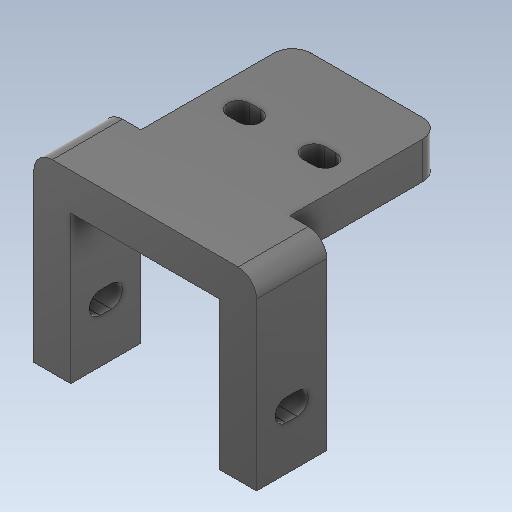
# Autodesk Inventor part: 0008-10-032 Suport cadru si axa Z
Saved by Autodesk Inventor 2020 (Build 240168000, 168)
## iProperties
Created: 2021-03-06
Part Number: 0008-10-032 Suport cadru si axa Z
Material: ABS Plastic
Document SubType Name: Modeling
Designer: Iulian Bors
Density: 1.06 g/cm^3
Appearance: Smooth - White
Mass: 43.4789 g
Surface Area: 130.984 cm^2
Volume: 41.0179 cm^3
Description: Suport cadru
Author: Iulian Bors
Subject: 032
Autodesk Inventor part; units mm, degrees
ref_plane "YZ Plane" through (0, 0, 0) normal (1, 0, 0) x (0, 1, 0)
ref_plane "XZ Plane" through (0, 0, 0) normal (0, 1, 0) x (-1, 0, 0)
ref_plane "XY Plane" through (0, 0, 0) normal (0, 0, 1) x (1, 0, 0)
sketch "Sketch1" plane through (0, 0, 0) normal (0, 0, 1) x (1, 0, 0)
  line L0 (-20.15, 20) -> (20.15, 20)
  line L1 (20.15, 20) -> (20.15, -20)
  line L2 (20.15, -20) -> (-20.15, -20)
  line L3 (-20.15, -20) -> (-20.15, 20)
  line L4 (30.15, 30) -> (-30.15, 30)
  line L5 (-30.15, 30) -> (-30.15, -30)
  line L6 (-30.15, -30) -> (30.15, -30)
  line L7 (30.15, -30) -> (30.15, 30)
  line L8 (-20.15, -20) -> (-30.15, -20)
  line L9 (20.15, -20) -> (30.15, -20)
  point P0 (0, 0)
  point P1 (0, 20)
  point P2 (-20.15, 0)
  dimension "d0" = 40.3
  dimension "d1" = 40
  dimension "d2" = 10
  constraints: 20 end point, 5 equal length, 3 perpendicular, 2 midpoint, 2 point on line, 1 horizontal, 1 horizontal alignment, 1 vertical alignment, 3 other
  measures "d0" distance of L0.start L0.end
  measures "d1" distance of L2.end L0.start
  measures "d2" distance between parallel lines of L0 L4
extrude "Extrusion1" add sketch "Sketch1" along normal blind 60 contours L3 L8 L5 L4 L7 L9 L1 L0
sketch "Sketch3" plane through (30.15, -20, 0) normal (1, 0, 0) x (0, 0, -1)
  line L0 (-41, 40) -> (0, 40)
  line L1 (0, 40) -> (0, 0)
  line L2 (0, 0) -> (-41, 0)
  line L3 (-41, 0) -> (-41, 40)
  line L4 (-60, 0) -> (-60, 50) projected
  line L5 (0, 0) -> (-60, 0) projected
  line L6 (0, 50) -> (-60, 50) projected
  line L7 (0, 0) -> (0, 50) projected
  point P0 (0, 20)
  dimension "d5" = 19
  dimension "d6" = 10
  constraints: 8 end point, 2 collinear, 2 parallel, 1 horizontal, 1 perpendicular
  measures "d5" distance between parallel lines of L3 L4
  measures "d6" distance between parallel lines of L0 L6
extrude "Extrusion2" cut sketch "Sketch3" against normal through all contours L0 L1 L2 L3
sketch "Sketch5" plane through (-30.15, 20, 0) normal (0, -1, 0) x (1, 0, 0)
  line L0 (60.3, 41) -> (50.3, 41)
  line L1 (50.3, 41) -> (50.3, 0)
  line L2 (50.3, 0) -> (60.3, 0)
  line L3 (60.3, 0) -> (60.3, 41)
  line L4 (60.3, 41) -> (60.3, 0) projected
  line L5 (0, 0) -> (60.3, 0) projected
  line L6 (60.3, 41) -> (50.3, 41) projected
  line L7 (50.3, 41) -> (50.3, 60) projected
  point P0 (30.15, 0)
  constraints: 8 end point, 4 collinear, 2 parallel, 1 horizontal, 1 perpendicular
extrude "Extrusion4" cut sketch "Sketch5" against normal through all
mirror "Mirror1" about plane through (0, 0, 0) normal (1, 0, 0) of "Extrusion4"
fillet "Fillet1" radius 5 4 edges at (-30.15, 30, 50.5) (30.15, 30, 50.5) (-20.15, 25, 0) (20.15, 25, 0)
sketch "Sketch9" plane through (30.15, -20, 60) normal (1, 0, 0) x (0, 0, -1)
  line L0 (8, 15) -> (11, 15) construction
  line L1 (8, 12) -> (11, 12)
  line L2 (11, 18) -> (8, 18)
  arc A0 (8, 18) -> (8, 12) centre (8, 15) ccw
  arc A1 (11, 12) -> (11, 18) centre (11, 15) ccw
  line L3 (19, 0) -> (0, 0) projected
  point P0 (60, 20)
  point P1 (9.5, 15)
  point P2 (9.5, 0)
  dimension "d34" = 3
  dimension "d35" = 6
  dimension "d36" = 15
  constraints: 8 end point, 4 point on circle, 4 tangent, 2 centre point, 2 midpoint, 1 horizontal, 1 parallel, 1 vertical alignment
  measures "d34" distance of L0.start L0.end
  measures "d35" diameter of A1
  measures "d36" distance from line of L3 point (9.5, 15)
extrude "Extrusion5" cut sketch "Sketch9" against normal through all
sketch "Sketch10" plane through (-15.15, 30, 0) normal (0, 1, 0) x (1, 0, 0)
  line L0 (3.5, -23) -> (6.5, -23) construction
  line L1 (3.5, -26) -> (6.5, -26)
  line L2 (6.5, -20) -> (3.5, -20)
  arc A0 (3.5, -20) -> (3.5, -26) centre (3.5, -23) ccw
  arc A1 (6.5, -26) -> (6.5, -20) centre (6.5, -23) ccw
  line L3 (23.8, -23) -> (26.8, -23) construction
  line L4 (23.8, -26) -> (26.8, -26)
  line L5 (26.8, -20) -> (23.8, -20)
  arc A2 (23.8, -20) -> (23.8, -26) centre (23.8, -23) ccw
  arc A3 (26.8, -26) -> (26.8, -20) centre (26.8, -23) ccw
  line L6 (-5, -5) -> (-5, -41) projected
  line L7 (35.3, -41) -> (35.3, -5) projected
  point P0 (15.15, 0)
  point P1 (5, -23)
  point P2 (25.3, -23)
  point P3 (-5, -23)
  dimension "d39" = 3
  dimension "d40" = 6
  dimension "d41" = 10
  dimension "d42" = 10
  constraints: 16 end point, 8 point on circle, 8 tangent, 4 centre point, 3 midpoint, 2 horizontal alignment, 2 parallel, 1 collinear, 1 equal radius, 1 horizontal, 1 perpendicular
  measures "d39" distance of L0.start L0.end
  measures "d40" diameter of A1
  measures "d41" distance from line of point (5, -23) L6
  measures "d42" distance from line of L7 point (25.3, -23)
extrude "Extrusion6" cut sketch "Sketch10" against normal through all
body "Solid1"
